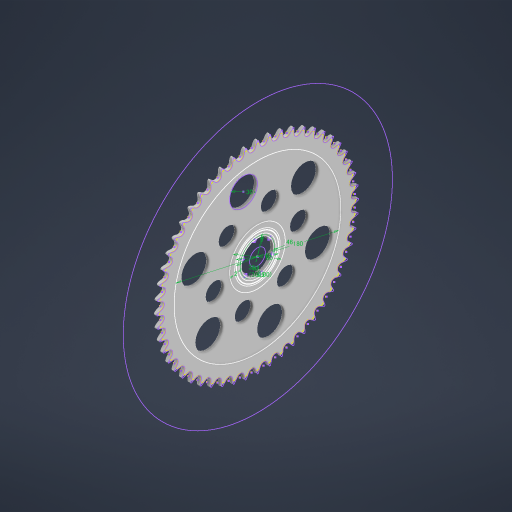
# Autodesk Inventor part: KANA40A52D17_6-D25_PCD124.6(H 7 D 0/+0.1 25 N/A)
Saved by Autodesk Inventor 2024.3 (Build 283343000, 343)
## iProperties
Category: PARTsolutions
Company: KANA
Created: 2025-03-03
Part Number: KANA40A52D17_6-D25_PCD124.6(H 7 D 0/+0.1 25 N/A)
Material: Generic
Catalog Web Link: www.cadenas.de
Description: 40A_semiF-Mounting holes
Vendor: KANA
Document SubType Name: Modeling
Designer: psAdmin
Manufacturer: KANA
Mass: 221.154 g
Surface Area: 728.752 cm^2
Volume: 221.154 cm^3
Density: 1 g/cm^3
Appearance: PSOLRGB-175-175-175
PSOL_IDENT_0: {$CADENAS_DATA/23d-libs/kana/sprockets/chain_no_40/un_finished_sprcoket_steel/a_type/40a_semi_f.prj}
PSOL_IDENT_1: ,274 {VTYP=3D},{NB=KANA40A52D17_6-D25_PCD124.6(H 7 D 0/+0.1 25 N/A)},{LINA=KANA40A52D17_6-D25_PCD124
PSOL_IDENT_2: .6},{NN=40A_semiF},{DATE=27.06.2023 01:46:20},{GEOMDATE=02.10.2020 05:05:43},{VERSION=},{LINEID=430}
PSOL_IDENT_3: ,{WBVAR=SD,SDAS,SDAC,NOH,TOH,HD,HDAV,TD,PCD,SURFT},{WBNUMERIC=SD,SDAC,HD,PCD}  {NB=KANA40A52D17_6-D2
PSOL_IDENT_4: 5_PCD124.6(H 7 D 0/+0.1 25 N/A)},{LINA=KANA40A52D17_6-D25_PCD124.6},{KT=DUMMY},{ORDERNO=KANA40A52D17
PSOL_IDENT_5: _6-D25_PCD124.6},{TYPE=40A},{NOT=52},{NOTX=52.000},{DP=210.34},{DC=202.39},{DC2=202.39},{DO=218},{H=
PSOL_IDENT_6: 5.9},{T=7.2},{DR=7.950},{MAT=None},{MATC=},{SD=17.0},{SDMIN=17.000},{SDMAX=190.6},{SDAS=H},{SDAC=7},
PSOL_IDENT_7: {SDACALG=7,6,8,9,10},{SDAV=0/+18},{SDAVMM=0/+0.018},{HDX=80.000},{PCDMT=51.500},{NOH=6},{NOHALG=<'','
PSOL_IDENT_8: No symbol : No'>,'1','1','2','2','3','3','4','4','5','5','6','6'},{NOHNUMB=6},{TOH=D},{TOHALG='D','D
PSOL_IDENT_9: : Drill hole','TC','TC : Tapped hole (Coarse screw)','TF','TF : Tapped hole (Fine pitch)'},{HD=25.0
PSOL_IDENT_10: },{HDALG=[4:25/0.1]},{HDMIN=4.0},{HDMAX=25.000},{HDAS= 'H', 'H', 'D', 'D', 'E', 'E', 'F', 'F', 'G', '
PSOL_IDENT_11: G', 'Js', 'Js', 'K'  , 'K', 'M', 'M', 'N', 'N'},{HDAC=$HDACALG.},{HDACALG=0},{HDAV=0/+0.1},{HDAVX=  '
PSOL_IDENT_12: +77,+50','+93,+50','+120,+50','+50,+32','+59,+32','+75,+32','+27,+16','+34,+16','+43,+16','+17,+6','
PSOL_IDENT_13: +24,+6','0, +11','0, +18','0, +27','0, +43','0, +70','-5.5,+5.5','-9,+9','-9, +2','-12, +6','-4,-15'
PSOL_IDENT_14: ,'-18, 0','-9,-20','-5,-23','-15,-26','-11, -29'     },{HDAVX2='0/+0.1','0/+0.2'},{HDAVMM=+0.050/+0.
PSOL_IDENT_15: 077},{TD=N/A},{TDALG='N/A','N/A'},{TDNDMNUMB=4},{TDKDMNUMB=3.242},{TDPNUMB=0.7},{PCD=124.6},{PCDALG=
PSOL_IDENT_16: <159.6>,[58:159.6/0.1]},{PCDMIN=58.0},{PCDMAX=159.6},{SURFT=},{NOHNB=_6},{HDNB=-D25},{TDNB=},{PCDNB=
PSOL_IDENT_17: _PCD124.6},{SURFTNB=},{TOHALGN=-D25},{DCX2=0},{CAUTION=The tooth profile in the CAD models differ fr
PSOL_IDENT_18: om the actual shape.}
NB: KANA40A52D17_6-D25_PCD124.6(H 7 D 0/+0.1 25 N/A)
NN: 40A_semiF
NT: Mounting holes
NBSYN: KANA40A$NOT.D$SD._$NOH.$TOHALGN._PCD$PCD.$SURFTNB.($SDAS. $SDAC. $TOH. $HDAV. $HD. $TD.)
LINA: KANA40A52D17_6-D25_PCD124.6
CATALOG: KANA
TYPE: 40A
NOT: 52
DP: 210.34
DC: 202.39
DC2: 202.39
DO: 218
T: 7.2
SD: 17
SDAS: H
SDAC: 7
SDAV: 0/+18
NOH: 6
TOH: D : Drill hole
HD: 25
HDAV: 0/+0.1
TD: N/A
PCD: 124.6
SURFT: No symbol : No
CAUTION: The tooth profile in the CAD models differ from the actual shape.
SUPPLIER: KANA
ARTICLENO: KANA40A52D17_6-D25_PCD124.6(H 7 D 0/+0.1 25 N/A)
BOMINFO: KANA40A52D17_6-D25_PCD124.6
CREATOR: CADENAS GmbH
Title: KANA40A52D17_6-D25_PCD124.6
Author: Cadenas PARTsolutions
Comments: Mounting holes
Autodesk Inventor part; units mm, degrees
ref_plane "YZ Plane" through (0, 0, 0) normal (1, 0, 0) x (0, 1, 0)
ref_plane "XZ Plane" through (0, 0, 0) normal (0, 1, 0) x (-1, 0, 0)
ref_plane "XY Plane" through (0, 0, 0) normal (0, 0, 1) x (1, 0, 0)
sketch "Sketch_1" plane through (0, 0, 0) normal (0, 0, 1) x (1, 0, 0)
  line L0 (7.2, 0) -> (0, 0)
  line L1 (0, 8.5) -> (3.2, 8.5)
  line L2 (3.2, 8.5) -> (3.2, 105.8394)
  arc A0 (3.2, 105.8394) -> (2.2899, 109) centre (-4.7294, 105.2675) ccw
  line L3 (2.2899, 109) -> (0.7899, 109)
  arc A1 (0.7899, 109) -> (0, 105.8394) centre (7.9441, 105.5329) ccw
  line L4 (0, 105.8394) -> (0, 8.5)
  dimension "d16" = 1.5
  dimension "d17" = 3.2
  constraints: 10 end point, 4 point on circle, 3 parallel, 2 centre point
  measures "d16" distance of L3.end L3.start
  measures "d17" distance of L4.start L2.end
revolve "Revolution1" add sketch "Sketch_1" angle 360 about axis through (7.2, 0, 0) along (1, 0, 0)
sketch "Sketch_2" plane through (3.6, 0, 0) normal (1, 0, 0) x (0, 0, -1)
  circle A0 centre (0, 0) radius 145.3333
  arc A1 (-108.9989, 0.5) -> (-108.9989, -0.5) centre (0, 0) ccw
  line L0 (-108.9989, -0.5) -> (-103.5248, -2.6502)
  arc A2 (-103.0895, -9.8477) -> (-103.5248, -2.6502) centre (-104.9781, -6.35) ccw
  line L1 (-103.0895, -9.8477) -> (-108.2644, -12.642)
  arc A3 (-108.2644, -12.642) -> (-108.1439, -13.6347) centre (0, 0) ccw
  line L2 (-108.1439, -13.6347) -> (-102.4506, -15.1094)
  arc A4 (-101.1508, -22.2019) -> (-102.4506, -15.1094) centre (-103.4473, -18.9574) ccw
  line L3 (-101.1508, -22.2019) -> (-105.9512, -25.5997)
  arc A5 (-105.9512, -25.5997) -> (-105.7119, -26.5706) centre (0, 0) ccw
  line L4 (-105.7119, -26.5706) -> (-99.8824, -27.3483)
  arc A6 (-97.7372, -34.2324) -> (-99.8824, -27.3483) centre (-100.408, -31.2884) ccw
  line L5 (-97.7372, -34.2324) -> (-102.093, -38.184)
  arc A7 (-102.093, -38.184) -> (-101.7384, -39.119) centre (0, 0) ccw
  line L6 (-101.7384, -39.119) -> (-95.8576, -39.1884)
  arc A8 (-92.8983, -45.7638) -> (-95.8576, -39.1884) centre (-95.9045, -43.1631) ccw
  line L7 (-92.8983, -45.7638) -> (-96.7461, -50.2116)
  arc A9 (-96.7461, -50.2116) -> (-96.2813, -51.097) centre (0, 0) ccw
  line L8 (-96.2813, -51.097) -> (-90.4351, -50.457)
  arc A10 (-86.7048, -56.6277) -> (-90.4351, -50.457) centre (-90.0025, -54.4084) ccw
  line L9 (-86.7048, -56.6277) -> (-89.9883, -61.5069)
  arc A11 (-89.9883, -61.5069) -> (-89.4203, -62.3299) centre (0, 0) ccw
  line L10 (-89.4203, -62.3299) -> (-83.6938, -60.9899)
  arc A12 (-79.2469, -66.666) -> (-83.6938, -60.9899) centre (-82.7881, -64.8603) ccw
  line L11 (-79.2469, -66.666) -> (-81.9184, -71.9054)
  arc A13 (-81.9184, -71.9054) -> (-81.2553, -72.6539) centre (0, 0) ccw
  line L12 (-81.2553, -72.6539) -> (-75.732, -70.6334)
  arc A14 (-70.6334, -75.732) -> (-75.732, -70.6334) centre (-74.3664, -74.3664) ccw
  line L13 (-70.6334, -75.732) -> (-72.6539, -81.2553)
  arc A15 (-72.6539, -81.2553) -> (-71.9054, -81.9184) centre (0, 0) ccw
  line L14 (-71.9054, -81.9184) -> (-66.666, -79.2469)
  arc A16 (-60.9899, -83.6938) -> (-66.666, -79.2469) centre (-64.8603, -82.7881) ccw
  line L15 (-60.9899, -83.6938) -> (-62.3299, -89.4203)
  arc A17 (-62.3299, -89.4203) -> (-61.5069, -89.9883) centre (0, 0) ccw
  line L16 (-61.5069, -89.9883) -> (-56.6277, -86.7048)
  arc A18 (-50.457, -90.4351) -> (-56.6277, -86.7048) centre (-54.4084, -90.0025) ccw
  line L17 (-50.457, -90.4351) -> (-51.097, -96.2813)
  arc A19 (-51.097, -96.2813) -> (-50.2116, -96.7461) centre (0, 0) ccw
  line L18 (-50.2116, -96.7461) -> (-45.7638, -92.8983)
  arc A20 (-39.1884, -95.8576) -> (-45.7638, -92.8983) centre (-43.1631, -95.9045) ccw
  line L19 (-39.1884, -95.8576) -> (-39.119, -101.7384)
  arc A21 (-39.119, -101.7384) -> (-38.184, -102.093) centre (0, 0) ccw
  line L20 (-38.184, -102.093) -> (-34.2324, -97.7372)
  arc A22 (-27.3483, -99.8824) -> (-34.2324, -97.7372) centre (-31.2884, -100.408) ccw
  line L21 (-27.3483, -99.8824) -> (-26.5706, -105.7119)
  arc A23 (-26.5706, -105.7119) -> (-25.5997, -105.9512) centre (0, 0) ccw
  line L22 (-25.5997, -105.9512) -> (-22.2019, -101.1508)
  arc A24 (-15.1094, -102.4506) -> (-22.2019, -101.1508) centre (-18.9574, -103.4473) ccw
  line L23 (-15.1094, -102.4506) -> (-13.6347, -108.1439)
  arc A25 (-13.6347, -108.1439) -> (-12.642, -108.2644) centre (0, 0) ccw
  line L24 (-12.642, -108.2644) -> (-9.8477, -103.0895)
  arc A26 (-2.6502, -103.5248) -> (-9.8477, -103.0895) centre (-6.35, -104.9781) ccw
  line L25 (-2.6502, -103.5248) -> (-0.5, -108.9989)
  arc A27 (-0.5, -108.9989) -> (0.5, -108.9989) centre (0, 0) ccw
  line L26 (0.5, -108.9989) -> (2.6502, -103.5248)
  arc A28 (9.8477, -103.0895) -> (2.6502, -103.5248) centre (6.35, -104.9781) ccw
  line L27 (9.8477, -103.0895) -> (12.642, -108.2644)
  arc A29 (12.642, -108.2644) -> (13.6347, -108.1439) centre (0, 0) ccw
  line L28 (13.6347, -108.1439) -> (15.1094, -102.4506)
  arc A30 (22.2019, -101.1508) -> (15.1094, -102.4506) centre (18.9574, -103.4473) ccw
  line L29 (22.2019, -101.1508) -> (25.5997, -105.9512)
  arc A31 (25.5997, -105.9512) -> (26.5706, -105.7119) centre (0, 0) ccw
  line L30 (26.5706, -105.7119) -> (27.3483, -99.8824)
  arc A32 (34.2324, -97.7372) -> (27.3483, -99.8824) centre (31.2884, -100.408) ccw
  line L31 (34.2324, -97.7372) -> (38.184, -102.093)
  arc A33 (38.184, -102.093) -> (39.119, -101.7384) centre (0, 0) ccw
  line L32 (39.119, -101.7384) -> (39.1884, -95.8576)
  arc A34 (45.7638, -92.8983) -> (39.1884, -95.8576) centre (43.1631, -95.9045) ccw
  line L33 (45.7638, -92.8983) -> (50.2116, -96.7461)
  arc A35 (50.2116, -96.7461) -> (51.097, -96.2813) centre (0, 0) ccw
  line L34 (51.097, -96.2813) -> (50.457, -90.4351)
  arc A36 (56.6277, -86.7048) -> (50.457, -90.4351) centre (54.4084, -90.0025) ccw
  line L35 (56.6277, -86.7048) -> (61.5069, -89.9883)
  arc A37 (61.5069, -89.9883) -> (62.3299, -89.4203) centre (0, 0) ccw
  line L36 (62.3299, -89.4203) -> (60.9899, -83.6938)
  arc A38 (66.666, -79.2469) -> (60.9899, -83.6938) centre (64.8603, -82.7881) ccw
  line L37 (66.666, -79.2469) -> (71.9054, -81.9184)
  arc A39 (71.9054, -81.9184) -> (72.6539, -81.2553) centre (0, 0) ccw
  line L38 (72.6539, -81.2553) -> (70.6334, -75.732)
  arc A40 (75.732, -70.6334) -> (70.6334, -75.732) centre (74.3664, -74.3664) ccw
  line L39 (75.732, -70.6334) -> (81.2553, -72.6539)
  arc A41 (81.2553, -72.6539) -> (81.9184, -71.9054) centre (0, 0) ccw
  line L40 (81.9184, -71.9054) -> (79.2469, -66.666)
  arc A42 (83.6938, -60.9899) -> (79.2469, -66.666) centre (82.7881, -64.8603) ccw
  line L41 (83.6938, -60.9899) -> (89.4203, -62.3299)
  arc A43 (89.4203, -62.3299) -> (89.9883, -61.5069) centre (0, 0) ccw
  line L42 (89.9883, -61.5069) -> (86.7048, -56.6277)
  arc A44 (90.4351, -50.457) -> (86.7048, -56.6277) centre (90.0025, -54.4084) ccw
  line L43 (90.4351, -50.457) -> (96.2813, -51.097)
  arc A45 (96.2813, -51.097) -> (96.7461, -50.2116) centre (0, 0) ccw
  line L44 (96.7461, -50.2116) -> (92.8983, -45.7638)
  arc A46 (95.8576, -39.1884) -> (92.8983, -45.7638) centre (95.9045, -43.1631) ccw
  line L45 (95.8576, -39.1884) -> (101.7384, -39.119)
  arc A47 (101.7384, -39.119) -> (102.093, -38.184) centre (0, 0) ccw
  line L46 (102.093, -38.184) -> (97.7372, -34.2324)
  arc A48 (99.8824, -27.3483) -> (97.7372, -34.2324) centre (100.408, -31.2884) ccw
  line L47 (99.8824, -27.3483) -> (105.7119, -26.5706)
  arc A49 (105.7119, -26.5706) -> (105.9512, -25.5997) centre (0, 0) ccw
  line L48 (105.9512, -25.5997) -> (101.1508, -22.2019)
  arc A50 (102.4506, -15.1094) -> (101.1508, -22.2019) centre (103.4473, -18.9574) ccw
  line L49 (102.4506, -15.1094) -> (108.1439, -13.6347)
  arc A51 (108.1439, -13.6347) -> (108.2644, -12.642) centre (0, 0) ccw
  line L50 (108.2644, -12.642) -> (103.0895, -9.8477)
  arc A52 (103.5248, -2.6502) -> (103.0895, -9.8477) centre (104.9781, -6.35) ccw
  line L51 (103.5248, -2.6502) -> (108.9989, -0.5)
  arc A53 (108.9989, -0.5) -> (108.9989, 0.5) centre (0, 0) ccw
  line L52 (108.9989, 0.5) -> (103.5248, 2.6502)
  arc A54 (103.0895, 9.8477) -> (103.5248, 2.6502) centre (104.9781, 6.35) ccw
  line L53 (103.0895, 9.8477) -> (108.2644, 12.642)
  arc A55 (108.2644, 12.642) -> (108.1439, 13.6347) centre (0, 0) ccw
  line L54 (108.1439, 13.6347) -> (102.4506, 15.1094)
  arc A56 (101.1508, 22.2019) -> (102.4506, 15.1094) centre (103.4473, 18.9574) ccw
  line L55 (101.1508, 22.2019) -> (105.9512, 25.5997)
  arc A57 (105.9512, 25.5997) -> (105.7119, 26.5706) centre (0, 0) ccw
  line L56 (105.7119, 26.5706) -> (99.8824, 27.3483)
  arc A58 (97.7372, 34.2324) -> (99.8824, 27.3483) centre (100.408, 31.2884) ccw
  line L57 (97.7372, 34.2324) -> (102.093, 38.184)
  arc A59 (102.093, 38.184) -> (101.7384, 39.119) centre (0, 0) ccw
  line L58 (101.7384, 39.119) -> (95.8576, 39.1884)
  arc A60 (92.8983, 45.7638) -> (95.8576, 39.1884) centre (95.9045, 43.1631) ccw
  line L59 (92.8983, 45.7638) -> (96.7461, 50.2116)
  arc A61 (96.7461, 50.2116) -> (96.2813, 51.097) centre (0, 0) ccw
  line L60 (96.2813, 51.097) -> (90.4351, 50.457)
  arc A62 (86.7048, 56.6277) -> (90.4351, 50.457) centre (90.0025, 54.4084) ccw
  line L61 (86.7048, 56.6277) -> (89.9883, 61.5069)
  arc A63 (89.9883, 61.5069) -> (89.4203, 62.3299) centre (0, 0) ccw
  line L62 (89.4203, 62.3299) -> (83.6938, 60.9899)
  arc A64 (79.2469, 66.666) -> (83.6938, 60.9899) centre (82.7881, 64.8603) ccw
  line L63 (79.2469, 66.666) -> (81.9184, 71.9054)
  arc A65 (81.9184, 71.9054) -> (81.2553, 72.6539) centre (0, 0) ccw
  line L64 (81.2553, 72.6539) -> (75.732, 70.6334)
  arc A66 (70.6334, 75.732) -> (75.732, 70.6334) centre (74.3664, 74.3664) ccw
  line L65 (70.6334, 75.732) -> (72.6539, 81.2553)
  arc A67 (72.6539, 81.2553) -> (71.9054, 81.9184) centre (0, 0) ccw
  line L66 (71.9054, 81.9184) -> (66.666, 79.2469)
  arc A68 (60.9899, 83.6938) -> (66.666, 79.2469) centre (64.8603, 82.7881) ccw
  line L67 (60.9899, 83.6938) -> (62.3299, 89.4203)
  arc A69 (62.3299, 89.4203) -> (61.5069, 89.9883) centre (0, 0) ccw
  line L68 (61.5069, 89.9883) -> (56.6277, 86.7048)
  arc A70 (50.457, 90.4351) -> (56.6277, 86.7048) centre (54.4084, 90.0025) ccw
  line L69 (50.457, 90.4351) -> (51.097, 96.2813)
  arc A71 (51.097, 96.2813) -> (50.2116, 96.7461) centre (0, 0) ccw
  line L70 (50.2116, 96.7461) -> (45.7638, 92.8983)
  arc A72 (39.1884, 95.8576) -> (45.7638, 92.8983) centre (43.1631, 95.9045) ccw
  line L71 (39.1884, 95.8576) -> (39.119, 101.7384)
  arc A73 (39.119, 101.7384) -> (38.184, 102.093) centre (0, 0) ccw
  line L72 (38.184, 102.093) -> (34.2324, 97.7372)
  arc A74 (27.3483, 99.8824) -> (34.2324, 97.7372) centre (31.2884, 100.408) ccw
  line L73 (27.3483, 99.8824) -> (26.5706, 105.7119)
  arc A75 (26.5706, 105.7119) -> (25.5997, 105.9512) centre (0, 0) ccw
  line L74 (25.5997, 105.9512) -> (22.2019, 101.1508)
  arc A76 (15.1094, 102.4506) -> (22.2019, 101.1508) centre (18.9574, 103.4473) ccw
  line L75 (15.1094, 102.4506) -> (13.6347, 108.1439)
  arc A77 (13.6347, 108.1439) -> (12.642, 108.2644) centre (0, 0) ccw
  line L76 (12.642, 108.2644) -> (9.8477, 103.0895)
  arc A78 (2.6502, 103.5248) -> (9.8477, 103.0895) centre (6.35, 104.9781) ccw
  line L77 (2.6502, 103.5248) -> (0.5, 108.9989)
  arc A79 (0.5, 108.9989) -> (-0.5, 108.9989) centre (0, 0) ccw
  line L78 (-0.5, 108.9989) -> (-2.6502, 103.5248)
  arc A80 (-9.8477, 103.0895) -> (-2.6502, 103.5248) centre (-6.35, 104.9781) ccw
  line L79 (-9.8477, 103.0895) -> (-12.642, 108.2644)
  arc A81 (-12.642, 108.2644) -> (-13.6347, 108.1439) centre (0, 0) ccw
  line L80 (-13.6347, 108.1439) -> (-15.1094, 102.4506)
  arc A82 (-22.2019, 101.1508) -> (-15.1094, 102.4506) centre (-18.9574, 103.4473) ccw
  line L81 (-22.2019, 101.1508) -> (-25.5997, 105.9512)
  arc A83 (-25.5997, 105.9512) -> (-26.5706, 105.7119) centre (0, 0) ccw
  line L82 (-26.5706, 105.7119) -> (-27.3483, 99.8824)
  arc A84 (-34.2324, 97.7372) -> (-27.3483, 99.8824) centre (-31.2884, 100.408) ccw
  line L83 (-34.2324, 97.7372) -> (-38.184, 102.093)
  arc A85 (-38.184, 102.093) -> (-39.119, 101.7384) centre (0, 0) ccw
  line L84 (-39.119, 101.7384) -> (-39.1884, 95.8576)
  arc A86 (-45.7638, 92.8983) -> (-39.1884, 95.8576) centre (-43.1631, 95.9045) ccw
  line L85 (-45.7638, 92.8983) -> (-50.2116, 96.7461)
  arc A87 (-50.2116, 96.7461) -> (-51.097, 96.2813) centre (0, 0) ccw
  line L86 (-51.097, 96.2813) -> (-50.457, 90.4351)
  arc A88 (-56.6277, 86.7048) -> (-50.457, 90.4351) centre (-54.4084, 90.0025) ccw
  line L87 (-56.6277, 86.7048) -> (-61.5069, 89.9883)
  arc A89 (-61.5069, 89.9883) -> (-62.3299, 89.4203) centre (0, 0) ccw
  line L88 (-62.3299, 89.4203) -> (-60.9899, 83.6938)
  arc A90 (-66.666, 79.2469) -> (-60.9899, 83.6938) centre (-64.8603, 82.7881) ccw
  line L89 (-66.666, 79.2469) -> (-71.9054, 81.9184)
  arc A91 (-71.9054, 81.9184) -> (-72.6539, 81.2553) centre (0, 0) ccw
  line L90 (-72.6539, 81.2553) -> (-70.6334, 75.732)
  arc A92 (-75.732, 70.6334) -> (-70.6334, 75.732) centre (-74.3664, 74.3664) ccw
  line L91 (-75.732, 70.6334) -> (-81.2553, 72.6539)
  arc A93 (-81.2553, 72.6539) -> (-81.9184, 71.9054) centre (0, 0) ccw
  line L92 (-81.9184, 71.9054) -> (-79.2469, 66.666)
  arc A94 (-83.6938, 60.9899) -> (-79.2469, 66.666) centre (-82.7881, 64.8603) ccw
  line L93 (-83.6938, 60.9899) -> (-89.4203, 62.3299)
  arc A95 (-89.4203, 62.3299) -> (-89.9883, 61.5069) centre (0, 0) ccw
  line L94 (-89.9883, 61.5069) -> (-86.7048, 56.6277)
  arc A96 (-90.4351, 50.457) -> (-86.7048, 56.6277) centre (-90.0025, 54.4084) ccw
  line L95 (-90.4351, 50.457) -> (-96.2813, 51.097)
  arc A97 (-96.2813, 51.097) -> (-96.7461, 50.2116) centre (0, 0) ccw
  line L96 (-96.7461, 50.2116) -> (-92.8983, 45.7638)
  arc A98 (-95.8576, 39.1884) -> (-92.8983, 45.7638) centre (-95.9045, 43.1631) ccw
  line L97 (-95.8576, 39.1884) -> (-101.7384, 39.119)
  arc A99 (-101.7384, 39.119) -> (-102.093, 38.184) centre (0, 0) ccw
  line L98 (-102.093, 38.184) -> (-97.7372, 34.2324)
  arc A100 (-99.8824, 27.3483) -> (-97.7372, 34.2324) centre (-100.408, 31.2884) ccw
  line L99 (-99.8824, 27.3483) -> (-105.7119, 26.5706)
  arc A101 (-105.7119, 26.5706) -> (-105.9512, 25.5997) centre (0, 0) ccw
  line L100 (-105.9512, 25.5997) -> (-101.1508, 22.2019)
  arc A102 (-102.4506, 15.1094) -> (-101.1508, 22.2019) centre (-103.4473, 18.9574) ccw
  line L101 (-102.4506, 15.1094) -> (-108.1439, 13.6347)
  arc A103 (-108.1439, 13.6347) -> (-108.2644, 12.642) centre (0, 0) ccw
  line L102 (-108.2644, 12.642) -> (-103.0895, 9.8477)
  arc A104 (-103.5248, 2.6502) -> (-103.0895, 9.8477) centre (-104.9781, 6.35) ccw
  line L103 (-103.5248, 2.6502) -> (-108.9989, 0.5)
  constraints: 208 end point, 208 point on circle, 105 centre point
extrude "Extrusion1" cut sketch "Sketch_2" along normal mid plane 7.6
sketch "スケッチ4" plane through (3.2, 18.9574, -103.4473) normal (1, 0, 0) x (0, 0.180255, -0.9836199)
  line L0 (-1.9941, -8.896) -> (0.3565, -8.1331) projected
  arc A0 (0.3565, -8.1331) -> (0.5674, -4.646) centre (-105.17, 0) ccw projected
  line L1 (0.5674, -4.646) -> (-1.674, -3.6053) projected
  arc A1 (-1.674, 3.6053) -> (-1.674, -3.6053) centre (0, 0) ccw projected
  line L2 (-1.674, 3.6053) -> (0.5674, 4.646) projected
  arc A2 (0.5674, 4.646) -> (0.3565, 8.1331) centre (-105.17, 0) ccw projected
  line L3 (0.3565, 8.1331) -> (-1.9941, 8.896) projected
  arc A3 (-2.8632, 16.0541) -> (-1.9941, 8.896) centre (-0.7668, 12.6768) ccw projected
  line L4 (-2.8632, 16.0541) -> (-0.7636, 17.3574) projected
  arc A4 (-0.7636, 17.3574) -> (-1.3933, 20.7936) centre (-105.17, 0) ccw projected
  line L5 (-1.3933, 20.7936) -> (-3.8186, 21.2677) projected
  arc A5 (-5.5442, 28.2688) -> (-3.8186, 21.2677) centre (-3.056, 25.1688) ccw projected
  line L6 (-5.5442, 28.2688) -> (-3.617, 29.8157) projected
  arc A6 (-3.617, 29.8157) -> (-4.6563, 33.1509) centre (-105.17, 0) ccw projected
  line L7 (-4.6563, 33.1509) -> (-7.1211, 33.3292) projected
  arc A7 (-9.678, 40.0712) -> (-7.1211, 33.3292) centre (-6.8343, 37.2938) ccw projected
  line L8 (-9.678, 40.0712) -> (-7.9513, 41.8391) projected
  arc A8 (-7.9513, 41.8391) -> (-9.3851, 45.0247) centre (-105.17, 0) ccw projected
  line L9 (-9.3851, 45.0247) -> (-11.8534, 44.9046) projected
  arc A9 (-15.2043, 51.2893) -> (-11.8534, 44.9046) centre (-12.0466, 48.8749) ccw projected
  line L10 (-15.2043, 51.2893) -> (-13.7033, 53.2525) projected
  arc A10 (-13.7033, 53.2525) -> (-15.5106, 56.2421) centre (-105.17, 0) ccw projected
  line L11 (-15.5106, 56.2421) -> (-17.9464, 55.8253) projected
  arc A11 (-22.0425, 61.7595) -> (-17.9464, 55.8253) centre (-18.6168, 59.7434) ccw projected
  line L12 (-22.0425, 61.7595) -> (-20.7891, 63.8893) projected
  arc A12 (-20.7891, 63.8893) -> (-22.9435, 66.6392) centre (-105.17, 0) ccw projected
  line L13 (-22.9435, 66.6392) -> (-25.3114, 65.9319) projected
  arc A13 (-30.0929, 71.3291) -> (-25.3114, 65.9319) centre (-26.4491, 69.7406) ccw projected
  line L14 (-30.0929, 71.3291) -> (-29.1053, 73.5945) projected
  arc A14 (-29.1053, 73.5945) -> (-31.5755, 76.0647) centre (-105.17, 0) ccw projected
  line L15 (-31.5755, 76.0647) -> (-33.8409, 75.0771) projected
  arc A15 (-39.2381, 79.8586) -> (-33.8409, 75.0771) centre (-35.4294, 78.7209) ccw projected
  line L16 (-39.2381, 79.8586) -> (-38.5308, 82.2265) projected
  arc A16 (-38.5308, 82.2265) -> (-41.2807, 84.3809) centre (-105.17, 0) ccw projected
  line L17 (-41.2807, 84.3809) -> (-43.4105, 83.1275) projected
  arc A17 (-49.3447, 87.2236) -> (-43.4105, 83.1275) centre (-45.4266, 86.5532) ccw projected
  line L18 (-49.3447, 87.2236) -> (-48.9279, 89.6594) projected
  arc A18 (-48.9279, 89.6594) -> (-51.9175, 91.4667) centre (-105.17, 0) ccw projected
  line L19 (-51.9175, 91.4667) -> (-53.8807, 89.9657) projected
  arc A19 (-60.2654, 93.3166) -> (-53.8807, 89.9657) centre (-56.2951, 93.1234) ccw projected
  line L20 (-60.2654, 93.3166) -> (-60.1453, 95.7849) projected
  arc A20 (-60.1453, 95.7849) -> (-63.3309, 97.2187) centre (-105.17, 0) ccw projected
  line L21 (-63.3309, 97.2187) -> (-65.0988, 95.492) projected
  arc A21 (-71.8408, 98.0489) -> (-65.0988, 95.492) centre (-67.8762, 98.3357) ccw projected
  line L22 (-71.8408, 98.0489) -> (-72.0191, 100.5137) projected
  arc A22 (-72.0191, 100.5137) -> (-75.3543, 101.553) centre (-105.17, 0) ccw projected
  line L23 (-75.3543, 101.553) -> (-76.9012, 99.6258) projected
  arc A23 (-83.9023, 101.3514) -> (-76.9012, 99.6258) centre (-80.0012, 102.114) ccw projected
  line L24 (-83.9023, 101.3514) -> (-84.3764, 103.7767) projected
  arc A24 (-84.3764, 103.7767) -> (-87.8126, 104.4064) centre (-105.17, 0) ccw projected
  line L25 (-87.8126, 104.4064) -> (-89.1159, 102.3068) projected
  arc A25 (-96.274, 103.1759) -> (-89.1159, 102.3068) centre (-92.4932, 104.4032) ccw projected
  line L26 (-96.274, 103.1759) -> (-97.0369, 105.5265) projected
  arc A26 (-97.0369, 105.5265) -> (-100.524, 105.7374) centre (-105.17, 0) ccw projected
  line L27 (-100.524, 105.7374) -> (-101.5647, 103.496) projected
  arc A27 (-108.7753, 103.496) -> (-101.5647, 103.496) centre (-105.17, 105.17) ccw projected
  line L28 (-108.7753, 103.496) -> (-109.816, 105.7374) projected
  arc A28 (-109.816, 105.7374) -> (-113.3031, 105.5265) centre (-105.17, 0) ccw projected
  line L29 (-113.3031, 105.5265) -> (-114.066, 103.1759) projected
  arc A29 (-121.2241, 102.3068) -> (-114.066, 103.1759) centre (-117.8468, 104.4032) ccw projected
  line L30 (-121.2241, 102.3068) -> (-122.5274, 104.4064) projected
  arc A30 (-122.5274, 104.4064) -> (-125.9636, 103.7767) centre (-105.17, 0) ccw projected
  line L31 (-125.9636, 103.7767) -> (-126.4377, 101.3514) projected
  arc A31 (-133.4388, 99.6258) -> (-126.4377, 101.3514) centre (-130.3388, 102.114) ccw projected
  line L32 (-133.4388, 99.6258) -> (-134.9857, 101.553) projected
  arc A32 (-134.9857, 101.553) -> (-138.3209, 100.5137) centre (-105.17, 0) ccw projected
  line L33 (-138.3209, 100.5137) -> (-138.4992, 98.0489) projected
  arc A33 (-145.2412, 95.492) -> (-138.4992, 98.0489) centre (-142.4638, 98.3357) ccw projected
  line L34 (-145.2412, 95.492) -> (-147.0091, 97.2187) projected
  arc A34 (-147.0091, 97.2187) -> (-150.1947, 95.7849) centre (-105.17, 0) ccw projected
  line L35 (-150.1947, 95.7849) -> (-150.0746, 93.3166) projected
  arc A35 (-156.4593, 89.9657) -> (-150.0746, 93.3166) centre (-154.0449, 93.1234) ccw projected
  line L36 (-156.4593, 89.9657) -> (-158.4225, 91.4667) projected
  arc A36 (-158.4225, 91.4667) -> (-161.4121, 89.6594) centre (-105.17, 0) ccw projected
  line L37 (-161.4121, 89.6594) -> (-160.9953, 87.2236) projected
  arc A37 (-166.9295, 83.1275) -> (-160.9953, 87.2236) centre (-164.9134, 86.5532) ccw projected
  line L38 (-166.9295, 83.1275) -> (-169.0593, 84.3809) projected
  arc A38 (-169.0593, 84.3809) -> (-171.8092, 82.2265) centre (-105.17, 0) ccw projected
  line L39 (-171.8092, 82.2265) -> (-171.1019, 79.8586) projected
  arc A39 (-176.4991, 75.0771) -> (-171.1019, 79.8586) centre (-174.9106, 78.7209) ccw projected
  line L40 (-176.4991, 75.0771) -> (-178.7645, 76.0647) projected
  arc A40 (-178.7645, 76.0647) -> (-181.2347, 73.5945) centre (-105.17, 0) ccw projected
  line L41 (-181.2347, 73.5945) -> (-180.2471, 71.3291) projected
  arc A41 (-185.0286, 65.9319) -> (-180.2471, 71.3291) centre (-183.8909, 69.7406) ccw projected
  line L42 (-185.0286, 65.9319) -> (-187.3965, 66.6392) projected
  arc A42 (-187.3965, 66.6392) -> (-189.5509, 63.8893) centre (-105.17, 0) ccw projected
  line L43 (-189.5509, 63.8893) -> (-188.2975, 61.7595) projected
  arc A43 (-192.3936, 55.8253) -> (-188.2975, 61.7595) centre (-191.7232, 59.7434) ccw projected
  line L44 (-192.3936, 55.8253) -> (-194.8294, 56.2421) projected
  arc A44 (-194.8294, 56.2421) -> (-196.6367, 53.2525) centre (-105.17, 0) ccw projected
  line L45 (-196.6367, 53.2525) -> (-195.1357, 51.2893) projected
  arc A45 (-198.4866, 44.9046) -> (-195.1357, 51.2893) centre (-198.2934, 48.8749) ccw projected
  line L46 (-198.4866, 44.9046) -> (-200.9549, 45.0247) projected
  arc A46 (-200.9549, 45.0247) -> (-202.3887, 41.8391) centre (-105.17, 0) ccw projected
  line L47 (-202.3887, 41.8391) -> (-200.662, 40.0712) projected
  arc A47 (-203.2189, 33.3292) -> (-200.662, 40.0712) centre (-203.5057, 37.2938) ccw projected
  line L48 (-203.2189, 33.3292) -> (-205.6837, 33.1509) projected
  arc A48 (-205.6837, 33.1509) -> (-206.723, 29.8157) centre (-105.17, 0) ccw projected
  line L49 (-206.723, 29.8157) -> (-204.7958, 28.2688) projected
  arc A49 (-206.5214, 21.2677) -> (-204.7958, 28.2688) centre (-207.284, 25.1688) ccw projected
  line L50 (-206.5214, 21.2677) -> (-208.9467, 20.7936) projected
  arc A50 (-208.9467, 20.7936) -> (-209.5764, 17.3574) centre (-105.17, 0) ccw projected
  line L51 (-209.5764, 17.3574) -> (-207.4768, 16.0541) projected
  arc A51 (-208.3459, 8.896) -> (-207.4768, 16.0541) centre (-209.5732, 12.6768) ccw projected
  line L52 (-208.3459, 8.896) -> (-210.6965, 8.1331) projected
  arc A52 (-210.6965, 8.1331) -> (-210.9074, 4.646) centre (-105.17, 0) ccw projected
  line L53 (-210.9074, 4.646) -> (-208.666, 3.6053) projected
  arc A53 (-208.666, -3.6053) -> (-208.666, 3.6053) centre (-210.34, 0) ccw projected
  line L54 (-208.666, -3.6053) -> (-210.9074, -4.646) projected
  arc A54 (-210.9074, -4.646) -> (-210.6965, -8.1331) centre (-105.17, 0) ccw projected
  line L55 (-210.6965, -8.1331) -> (-208.3459, -8.896) projected
  arc A55 (-207.4768, -16.0541) -> (-208.3459, -8.896) centre (-209.5732, -12.6768) ccw projected
  line L56 (-207.4768, -16.0541) -> (-209.5764, -17.3574) projected
  arc A56 (-209.5764, -17.3574) -> (-208.9467, -20.7936) centre (-105.17, 0) ccw projected
  line L57 (-208.9467, -20.7936) -> (-206.5214, -21.2677) projected
  arc A57 (-204.7958, -28.2688) -> (-206.5214, -21.2677) centre (-207.284, -25.1688) ccw projected
  line L58 (-204.7958, -28.2688) -> (-206.723, -29.8157) projected
  arc A58 (-206.723, -29.8157) -> (-205.6837, -33.1509) centre (-105.17, 0) ccw projected
  line L59 (-205.6837, -33.1509) -> (-203.2189, -33.3292) projected
  arc A59 (-200.662, -40.0712) -> (-203.2189, -33.3292) centre (-203.5057, -37.2938) ccw projected
  line L60 (-200.662, -40.0712) -> (-202.3887, -41.8391) projected
  arc A60 (-202.3887, -41.8391) -> (-200.9549, -45.0247) centre (-105.17, 0) ccw projected
  line L61 (-200.9549, -45.0247) -> (-198.4866, -44.9046) projected
  arc A61 (-195.1357, -51.2893) -> (-198.4866, -44.9046) centre (-198.2934, -48.8749) ccw projected
  line L62 (-195.1357, -51.2893) -> (-196.6367, -53.2525) projected
  arc A62 (-196.6367, -53.2525) -> (-194.8294, -56.2421) centre (-105.17, 0) ccw projected
  line L63 (-194.8294, -56.2421) -> (-192.3936, -55.8253) projected
  arc A63 (-188.2975, -61.7595) -> (-192.3936, -55.8253) centre (-191.7232, -59.7434) ccw projected
  line L64 (-188.2975, -61.7595) -> (-189.5509, -63.8893) projected
  arc A64 (-189.5509, -63.8893) -> (-187.3965, -66.6392) centre (-105.17, 0) ccw projected
  line L65 (-187.3965, -66.6392) -> (-185.0286, -65.9319) projected
  arc A65 (-180.2471, -71.3291) -> (-185.0286, -65.9319) centre (-183.8909, -69.7406) ccw projected
  line L66 (-180.2471, -71.3291) -> (-181.2347, -73.5945) projected
  arc A66 (-181.2347, -73.5945) -> (-178.7645, -76.0647) centre (-105.17, 0) ccw projected
  line L67 (-178.7645, -76.0647) -> (-176.4991, -75.0771) projected
  arc A67 (-171.1019, -79.8586) -> (-176.4991, -75.0771) centre (-174.9106, -78.7209) ccw projected
  line L68 (-171.1019, -79.8586) -> (-171.8092, -82.2265) projected
  arc A68 (-171.8092, -82.2265) -> (-169.0593, -84.3809) centre (-105.17, 0) ccw projected
  line L69 (-169.0593, -84.3809) -> (-166.9295, -83.1275) projected
  arc A69 (-160.9953, -87.2236) -> (-166.9295, -83.1275) centre (-164.9134, -86.5532) ccw projected
  line L70 (-160.9953, -87.2236) -> (-161.4121, -89.6594) projected
  arc A70 (-161.4121, -89.6594) -> (-158.4225, -91.4667) centre (-105.17, 0) ccw projected
  line L71 (-158.4225, -91.4667) -> (-156.4593, -89.9657) projected
  arc A71 (-150.0746, -93.3166) -> (-156.4593, -89.9657) centre (-154.0449, -93.1234) ccw projected
  line L72 (-150.0746, -93.3166) -> (-150.1947, -95.7849) projected
  arc A72 (-150.1947, -95.7849) -> (-147.0091, -97.2187) centre (-105.17, 0) ccw projected
  line L73 (-147.0091, -97.2187) -> (-145.2412, -95.492) projected
  arc A73 (-138.4992, -98.0489) -> (-145.2412, -95.492) centre (-142.4638, -98.3357) ccw projected
  line L74 (-138.4992, -98.0489) -> (-138.3209, -100.5137) projected
  arc A74 (-138.3209, -100.5137) -> (-134.9857, -101.553) centre (-105.17, 0) ccw projected
  line L75 (-134.9857, -101.553) -> (-133.4388, -99.6258) projected
  arc A75 (-126.4377, -101.3514) -> (-133.4388, -99.6258) centre (-130.3388, -102.114) ccw projected
  line L76 (-126.4377, -101.3514) -> (-125.9636, -103.7767) projected
  arc A76 (-125.9636, -103.7767) -> (-122.5274, -104.4064) centre (-105.17, 0) ccw projected
  line L77 (-122.5274, -104.4064) -> (-121.2241, -102.3068) projected
  arc A77 (-114.066, -103.1759) -> (-121.2241, -102.3068) centre (-117.8468, -104.4032) ccw projected
  line L78 (-114.066, -103.1759) -> (-113.3031, -105.5265) projected
  arc A78 (-113.3031, -105.5265) -> (-109.816, -105.7374) centre (-105.17, 0) ccw projected
  line L79 (-109.816, -105.7374) -> (-108.7753, -103.496) projected
  arc A79 (-101.5647, -103.496) -> (-108.7753, -103.496) centre (-105.17, -105.17) ccw projected
  line L80 (-101.5647, -103.496) -> (-100.524, -105.7374) projected
  arc A80 (-100.524, -105.7374) -> (-97.0369, -105.5265) centre (-105.17, 0) ccw projected
  line L81 (-97.0369, -105.5265) -> (-96.274, -103.1759) projected
  arc A81 (-89.1159, -102.3068) -> (-96.274, -103.1759) centre (-92.4932, -104.4032) ccw projected
  line L82 (-89.1159, -102.3068) -> (-87.8126, -104.4064) projected
  arc A82 (-87.8126, -104.4064) -> (-84.3764, -103.7767) centre (-105.17, 0) ccw projected
  line L83 (-84.3764, -103.7767) -> (-83.9023, -101.3514) projected
  arc A83 (-76.9012, -99.6258) -> (-83.9023, -101.3514) centre (-80.0012, -102.114) ccw projected
  line L84 (-76.9012, -99.6258) -> (-75.3543, -101.553) projected
  arc A84 (-75.3543, -101.553) -> (-72.0191, -100.5137) centre (-105.17, 0) ccw projected
  line L85 (-72.0191, -100.5137) -> (-71.8408, -98.0489) projected
  arc A85 (-65.0988, -95.492) -> (-71.8408, -98.0489) centre (-67.8762, -98.3357) ccw projected
  line L86 (-65.0988, -95.492) -> (-63.3309, -97.2187) projected
  arc A86 (-63.3309, -97.2187) -> (-60.1453, -95.7849) centre (-105.17, 0) ccw projected
  line L87 (-60.1453, -95.7849) -> (-60.2654, -93.3166) projected
  arc A87 (-53.8807, -89.9657) -> (-60.2654, -93.3166) centre (-56.2951, -93.1234) ccw projected
  line L88 (-53.8807, -89.9657) -> (-51.9175, -91.4667) projected
  arc A88 (-51.9175, -91.4667) -> (-48.9279, -89.6594) centre (-105.17, 0) ccw projected
  line L89 (-48.9279, -89.6594) -> (-49.3447, -87.2236) projected
  arc A89 (-43.4105, -83.1275) -> (-49.3447, -87.2236) centre (-45.4266, -86.5532) ccw projected
  line L90 (-43.4105, -83.1275) -> (-41.2807, -84.3809) projected
  arc A90 (-41.2807, -84.3809) -> (-38.5308, -82.2265) centre (-105.17, 0) ccw projected
  line L91 (-38.5308, -82.2265) -> (-39.2381, -79.8586) projected
  arc A91 (-33.8409, -75.0771) -> (-39.2381, -79.8586) centre (-35.4294, -78.7209) ccw projected
  line L92 (-33.8409, -75.0771) -> (-31.5755, -76.0647) projected
  arc A92 (-31.5755, -76.0647) -> (-29.1053, -73.5945) centre (-105.17, 0) ccw projected
  line L93 (-29.1053, -73.5945) -> (-30.0929, -71.3291) projected
  arc A93 (-25.3114, -65.9319) -> (-30.0929, -71.3291) centre (-26.4491, -69.7406) ccw projected
  line L94 (-25.3114, -65.9319) -> (-22.9435, -66.6392) projected
  arc A94 (-22.9435, -66.6392) -> (-20.7891, -63.8893) centre (-105.17, 0) ccw projected
  line L95 (-20.7891, -63.8893) -> (-22.0425, -61.7595) projected
  arc A95 (-17.9464, -55.8253) -> (-22.0425, -61.7595) centre (-18.6168, -59.7434) ccw projected
  line L96 (-17.9464, -55.8253) -> (-15.5106, -56.2421) projected
  arc A96 (-15.5106, -56.2421) -> (-13.7033, -53.2525) centre (-105.17, 0) ccw projected
  line L97 (-13.7033, -53.2525) -> (-15.2043, -51.2893) projected
  arc A97 (-11.8534, -44.9046) -> (-15.2043, -51.2893) centre (-12.0466, -48.8749) ccw projected
  line L98 (-11.8534, -44.9046) -> (-9.3851, -45.0247) projected
  arc A98 (-9.3851, -45.0247) -> (-7.9513, -41.8391) centre (-105.17, 0) ccw projected
  line L99 (-7.9513, -41.8391) -> (-9.678, -40.0712) projected
  arc A99 (-7.1211, -33.3292) -> (-9.678, -40.0712) centre (-6.8343, -37.2938) ccw projected
  line L100 (-7.1211, -33.3292) -> (-4.6563, -33.1509) projected
  arc A100 (-4.6563, -33.1509) -> (-3.617, -29.8157) centre (-105.17, 0) ccw projected
  line L101 (-3.617, -29.8157) -> (-5.5442, -28.2688) projected
  arc A101 (-3.8186, -21.2677) -> (-5.5442, -28.2688) centre (-3.056, -25.1688) ccw projected
  line L102 (-3.8186, -21.2677) -> (-1.3933, -20.7936) projected
  arc A102 (-1.3933, -20.7936) -> (-0.7636, -17.3574) centre (-105.17, 0) ccw projected
  line L103 (-0.7636, -17.3574) -> (-2.8632, -16.0541) projected
  arc A103 (-1.9941, -8.896) -> (-2.8632, -16.0541) centre (-0.7668, -12.6768) ccw projected
  circle A104 centre (-105.17, 0) radius 8.5 projected
  circle A105 centre (-105.17, 0) radius 8.5 projected
  line L104 (-105.1672, -17.55) -> (-105.1672, -15.55)
  arc A106 (-102.4172, -17.3328) -> (-107.9172, -17.3337) centre (-105.167, -18.5621) ccw
  line L105 (-107.9172, -17.0014) -> (-107.9172, -18.0986) construction
  line L106 (-102.4172, -18.0986) -> (-102.4172, -17.0014) construction
  line L107 (-107.9172, -18.0986) -> (-102.4172, -18.0986) construction
  line L108 (-107.9172, -17.0014) -> (-102.4172, -18.0986) construction
  line L109 (-102.4172, -17.0014) -> (-107.9172, -18.0986) construction
  line L110 (-102.4172, -17.0014) -> (-107.9172, -17.0014) construction
  arc A107 (-121.557, 6.2823) -> (-118.8078, 11.0459) centre (-121.2468, 9.2784) ccw
  arc A108 (-107.9228, 17.3328) -> (-102.4228, 17.3337) centre (-105.173, 18.5621) ccw
  arc A109 (-91.5358, 11.0504) -> (-88.785, 6.2877) centre (-89.0963, 9.2837) ccw
  arc A110 (-88.783, -6.2823) -> (-91.5322, -11.0459) centre (-89.0932, -9.2784) ccw
  arc A111 (-118.8042, -11.0504) -> (-121.555, -6.2877) centre (-121.2437, -9.2837) ccw
  circle A112 centre (-105.17, 0) radius 20
  circle A113 centre (-105.17, 0) radius 17.55
  circle A114 centre (-105.17, 0) radius 8.5
  circle A115 centre (-105.17, 0) radius 24.5
  circle A116 centre (-105.17, 0) radius 23
  circle A117 centre (-105.17, 0) radius 24.5
  circle A118 centre (-105.17, 0) radius 22.5
  point P0 (-118.6381, 7.7725)
  point P1 (-105.1728, 15.55)
  point P2 (-91.7047, 7.7775)
  point P3 (-91.7019, -7.7725)
  point P4 (-118.6353, -7.7775)
  point P5 (-91.5322, -11.0459)
  point P6 (-88.783, -6.2823)
  point P7 (-88.785, 6.2877)
  point P8 (-91.5358, 11.0504)
  point P9 (-102.4228, 17.3337)
  point P10 (-107.9228, 17.3328)
  point P11 (-118.8078, 11.0459)
  point P12 (-121.557, 6.2823)
  point P13 (-121.555, -6.2877)
  point P14 (-118.8042, -11.0504)
  dimension "d20" = 35.1
  dimension "d21" = 2
  dimension "d22" = 5.5
  dimension "d23" = 360
  dimension "d24" = 40
  dimension "d25" = 49
  dimension "d26" = 46
  dimension "d29" = 2
  constraints: 21 point on circle, 14 end point, 13 centre point, 9 coincident, 2 midpoint, 2 parallel, 2 point on line, 1 concentric, 1 horizontal, 1 perpendicular, 1 vertical, 31 other
  measures "d20" diameter of A113
  measures "d21" distance of L104.start L104.end
  measures "d22" distance of L107.end L105.end
  measures "d24" diameter of A112
  measures "d25" diameter of A115
  measures "d26" diameter of A116
  measures "d29" radial gap between concentric circles of A115 A118
extrude "押し出し2" cut sketch "スケッチ4" against normal through all contours A106 A113 A111 A107 A108 A109 A110
sketch "スケッチ5" plane through (3.2, 18.9574, -103.4473) normal (1, 0, 0) x (0, 0.180255, -0.9836199)
  circle A0 centre (-107.7065, 69.9311) radius 15
  circle A1 centre (-105.17, 0) radius 90
  circle A2 centre (-105.17, 0) radius 30
  dimension "d30" = 30
  dimension "d31" = 180
  dimension "d32" = 60
  constraints: 3 centre point, 2 coincident
  measures "d30" diameter of A0
  measures "d31" diameter of A1
  measures "d32" diameter of A2
extrude "押し出し3" cut sketch "スケッチ5" against normal blind 0.4
extrude "押し出し4" cut sketch "スケッチ5" against normal through all contours A0
pattern_circular "円形状パターン1" count 6 over 360 about axis through (3.2, 0, 0) along (-1, 0, 0) of "押し出し4"
sketch "スケッチ6" plane through (2.8, 0, 0) normal (1, 0, 0) x (0, 0, -1)
  circle A0 centre (-15.1004, 68.3284) radius 15 projected
  circle A1 centre (-66.7243, 21.0869) radius 15 projected
  line L0 (-66.7243, 21.0869) -> (-15.1004, 68.3284)
  circle A2 centre (-31.4807, 34.4011) radius 10
  point P0 (0, 0)
  dimension "d40" = 20
  constraints: 2 end point, 1 centre point
  measures "d40" diameter of A2
extrude "押し出し5" cut sketch "スケッチ6" against normal through all contours A2
pattern_circular "円形状パターン2" count 6 over 360 about axis through (3.2, 0, 0) along (-1, 0, 0) of "押し出し5"
body "Solid1"
